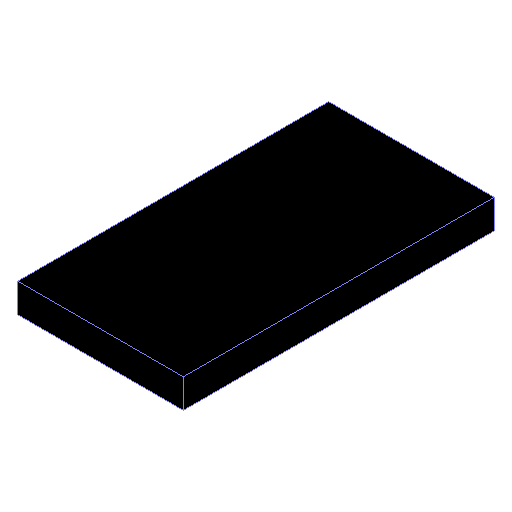
# Autodesk Inventor part: gps_black
Saved by Autodesk Inventor 2025.2 (Build 292293000, 293)
## iProperties
Created: 2025-03-31
Part Number: gps_black
Material: 일반
Document SubType Name: Modeling
Designer: jbhma
Density: 1 g/cm^3
Appearance: 기본값
Author: jbhma
Autodesk Inventor part; units mm, degrees
ref_plane "YZ Plane" through (0, 0, 0) normal (1, 0, 0) x (0, 1, 0)
ref_plane "XZ Plane" through (0, 0, 0) normal (0, 1, 0) x (-1, 0, 0)
ref_plane "XY Plane" through (0, 0, 0) normal (0, 0, 1) x (1, 0, 0)
sketch "스케치1" plane through (0, 0, 0) normal (0, 1, 0) x (-1, 0, 0)
  line L0 (0, 0) -> (-57, 0)
  line L1 (-57, 0) -> (-57, -107)
  line L2 (-57, -107) -> (0, -107)
  line L3 (0, -107) -> (0, 0)
  dimension "d0" = 57
  dimension "d1" = 107
  constraints: 8 end point, 2 parallel, 1 horizontal, 1 perpendicular
  measures "d0" distance of L2.end L1.end
  measures "d1" distance of L1.end L0.end
extrude "돌출1" add sketch "스케치1" along normal blind 10
